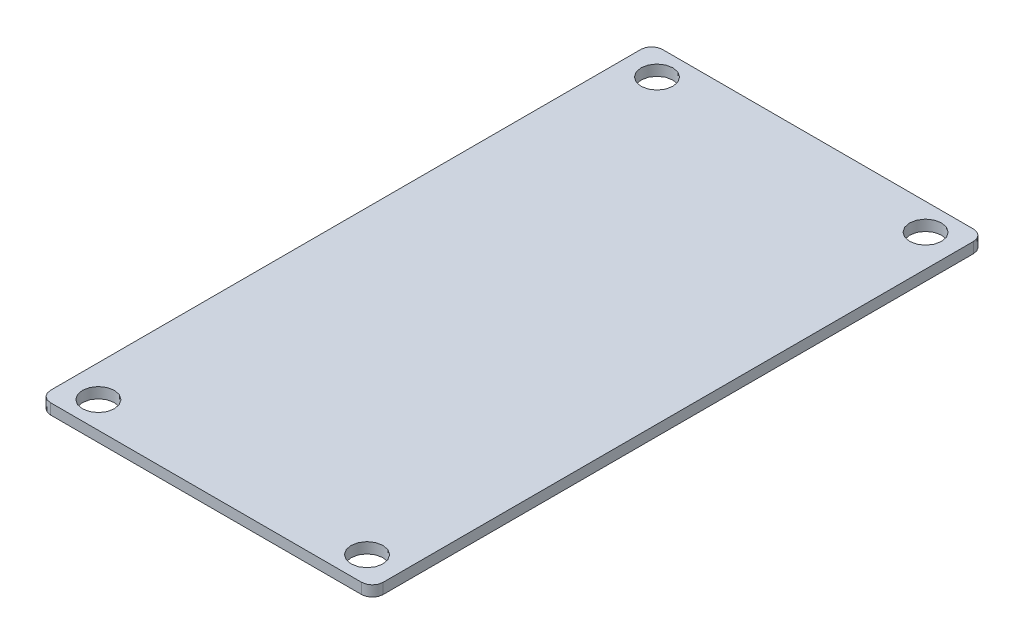
# Autodesk Inventor part: esp8266_footprint
Saved by Autodesk Inventor 2019 (Build 230136000, 136)
## iProperties
Created: 2019-04-09
Part Number: esp8266_footprint
Material: Generic
Document SubType Name: Modeling
Designer: jmc
Density: 1 g/cm^3
Appearance: Default
Author: jmc
Autodesk Inventor part; units mm, degrees
ref_plane "YZ Plane" through (0, 0, 0) normal (1, 0, 0) x (0, 1, 0)
ref_plane "XZ Plane" through (0, 0, 0) normal (0, 1, 0) x (-1, 0, 0)
ref_plane "XY Plane" through (0, 0, 0) normal (0, 0, 1) x (1, 0, 0)
sketch "Sketch1" plane through (0, 0, 0) normal (0, 0, 1) x (1, 0, 0)
  point P0 (0, 0)
sketch "Sketch2" plane through (0, 0, 0) normal (0, 1, 0) x (-1, 0, 0)
  line L0 (14.6, 28.7) -> (-14.6, 28.7)
  line L1 (-15.6, 27.7) -> (-15.6, -27.7)
  line L2 (-14.6, -28.7) -> (14.6, -28.7)
  line L3 (15.6, -27.7) -> (15.6, 27.7)
  line L4 (15.6, 28.7) -> (-15.6, -28.7) construction
  line L5 (-15.6, 28.7) -> (15.6, -28.7) construction
  arc A0 (15.6, 27.7) -> (14.6, 28.7) centre (14.6, 27.7) ccw
  arc A1 (-14.6, 28.7) -> (-15.6, 27.7) centre (-14.6, 27.7) ccw
  arc A2 (14.6, -28.7) -> (15.6, -27.7) centre (14.6, -27.7) ccw
  arc A3 (-15.6, -27.7) -> (-14.6, -28.7) centre (-14.6, -27.7) ccw
  circle A4 centre (12.6, 26.2) radius 1.5
  line L6 (0, 28.7) -> (0, -28.7) construction
  line L7 (15.6, 0) -> (-15.6, 0) construction
  circle A5 centre (12.6, -26.2) radius 1.5
  circle A6 centre (-12.6, 26.2) radius 1.5
  circle A7 centre (-12.6, -26.2) radius 1.5
  line L8 (1.792, 7.3985) -> (1.792, -6.1335) construction
  line L9 (1.792, -6.1335) -> (-36.4686, -6.1335) construction
  line L10 (-36.4686, -6.1335) -> (-36.4686, 7.3985) construction
  line L11 (-36.4686, 7.3985) -> (1.792, 7.3985) construction
  point P0 (0, 0)
  dimension "d0" = 31.2
  dimension "d1" = 57.4
  dimension "d2" = 1
  dimension "d3" = 3
  dimension "d4" = 3
  dimension "d5" = 2.5
  constraints: 16 end point, 8 centre point, 8 point on circle, 8 point on line, 8 tangent, 6 midpoint, 3 equal radius, 3 symmetric about line, 2 parallel, 1 horizontal, 1 perpendicular, 5 other
  measures "d0" distance of L5.end L4.end
  measures "d1" distance of L4.end L5.start
  measures "d2" radius of A0
  measures "d3" diameter of A4
  measures "d4" distance from line of L3 A4.centre
  measures "d5" distance from line of L0 A4.centre
extrude "Extrusion1" add sketch "Sketch2" along normal blind 1
body "Solid1"
